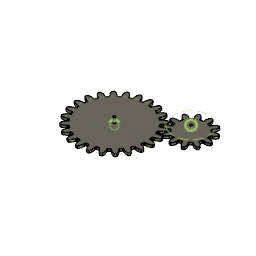
day5 joint and motion (Autodesk Fusion 360 design; units mm, degrees)
part number: 2026-04-16-20-59-54-327
description: Spur Gear; Module: 12.7; Num Teeth: 24; Pressure Angle: 20.0; Backlash: 0.00 mm
part number: 2026-04-16-21-00-13-750
description: Spur Gear; Module: 12.7; Num Teeth: 12; Pressure Angle: 20.0; Backlash: 0.00 mm
part number: 2026-04-16-21-00-25-707
part number: 2026-04-16-21-14-06-063
Autodesk Fusion 360 part; units mm, degrees
(part 1 of 2)
sketch "Base Circle" plane through (0, 0, 0) normal (0, 0, 1) x (1, 0, 0) in component "Spur Gear 24 teeth"
  circle A0 centre (0, 0) radius 137.7061
  circle A1 centre (0, 0) radius 5
extrude "Extrude1" add sketch "Base Circle" along normal blind 10 makes body 1 in component "Spur Gear 24 teeth"
sketch "Gear Tooth" plane through (0, 0, 0) normal (0, 0, 1) x (1, 0, 0) in component "Spur Gear 24 teeth"
  spline S0 degree 5 poles (142.7471, -11.4951) (142.8118, -11.5003) (142.9412, -11.5091) (143.1354, -11.5173) (143.3946, -11.5189) (143.7188, -11.5082) (144.0432, -11.4883) (144.3678, -11.4628) (144.6924, -11.4343) (145.0169, -11.4038) (145.3415, -11.3711) (145.666, -11.3355) (145.9905, -11.2961) (146.3148, -11.2522) (146.6391, -11.2039) (146.9633, -11.1516) (147.2873, -11.0957) (147.6112, -11.037) (147.935, -10.9757) (148.2586, -10.9121) (148.5821, -10.846) (148.9053, -10.7774) (149.2285, -10.7062) (149.5514, -10.6322) (149.8741, -10.5555) (150.1966, -10.4762) (150.5189, -10.3945) (150.8411, -10.3105) (151.1629, -10.2242) (151.4846, -10.1358) (151.806, -10.0451) (152.1272, -9.9523) (152.4482, -9.8574) (152.7689, -9.7602) (153.0893, -9.661) (153.4095, -9.5596) (153.7295, -9.4562) (154.0491, -9.3508) (154.3685, -9.2434) (154.6877, -9.1341) (155.0065, -9.0228) (155.325, -8.9096) (155.6433, -8.7946) (155.9613, -8.6776) (156.279, -8.5588) (156.5963, -8.4382) (156.9134, -8.3157) (157.2301, -8.1914) (157.5466, -8.0654) (157.8627, -7.9376) (158.1785, -7.808) (158.494, -7.6767) (158.8091, -7.5437) (159.1239, -7.409) (159.4384, -7.2727) (159.7525, -7.1346) (160.0663, -6.9949) (160.3798, -6.8535) (160.6929, -6.7105) (161.0056, -6.5659) (161.318, -6.4196) (161.63, -6.2718) (161.9417, -6.1224) (162.253, -5.9714) (162.5639, -5.8189) (162.8745, -5.6648) (163.1846, -5.5091) (163.4944, -5.352) (163.8038, -5.1933) (164.1128, -5.0331) (164.4215, -4.8714) (164.6681, -4.7409) (164.8528, -4.6423) (164.9759, -4.5763) (165.0375, -4.5432) knots 0 0 0 0 0 0 0.01428571 0.02857143 0.04285714 0.05714286 0.07142857 0.08571429 0.1 0.11428571 0.12857143 0.14285714 0.15714286 0.17142857 0.18571429 0.2 0.21428571 0.22857143 0.24285714 0.25714286 0.27142857 0.28571429 0.3 0.31428571 0.32857143 0.34285714 0.35714286 0.37142857 0.38571429 0.4 0.41428571 0.42857143 0.44285714 0.45714286 0.47142857 0.48571429 0.5 0.51428571 0.52857143 0.54285714 0.55714286 0.57142857 0.58571429 0.6 0.61428571 0.62857143 0.64285714 0.65714286 0.67142857 0.68571429 0.7 0.71428571 0.72857143 0.74285714 0.75714286 0.77142857 0.78571429 0.8 0.81428571 0.82857143 0.84285714 0.85714286 0.87142857 0.88571429 0.9 0.91428571 0.92857143 0.94285714 0.95714286 0.97142857 0.98571429 1 1 1 1 1 1
  spline S1 degree 5 poles (142.7471, 11.4951) (142.8118, 11.5003) (142.9412, 11.5091) (143.1354, 11.5173) (143.3946, 11.5189) (143.7188, 11.5082) (144.0432, 11.4883) (144.3678, 11.4628) (144.6924, 11.4343) (145.0169, 11.4038) (145.3415, 11.3711) (145.666, 11.3355) (145.9905, 11.2961) (146.3148, 11.2522) (146.6391, 11.2039) (146.9633, 11.1516) (147.2873, 11.0957) (147.6112, 11.037) (147.935, 10.9757) (148.2586, 10.9121) (148.5821, 10.846) (148.9053, 10.7774) (149.2285, 10.7062) (149.5514, 10.6322) (149.8741, 10.5555) (150.1966, 10.4762) (150.5189, 10.3945) (150.8411, 10.3105) (151.1629, 10.2242) (151.4846, 10.1358) (151.806, 10.0451) (152.1272, 9.9523) (152.4482, 9.8574) (152.7689, 9.7602) (153.0893, 9.661) (153.4095, 9.5596) (153.7295, 9.4562) (154.0491, 9.3508) (154.3685, 9.2434) (154.6877, 9.1341) (155.0065, 9.0228) (155.325, 8.9096) (155.6433, 8.7946) (155.9613, 8.6776) (156.279, 8.5588) (156.5963, 8.4382) (156.9134, 8.3157) (157.2301, 8.1914) (157.5466, 8.0654) (157.8627, 7.9376) (158.1785, 7.808) (158.494, 7.6767) (158.8091, 7.5437) (159.1239, 7.409) (159.4384, 7.2727) (159.7525, 7.1346) (160.0663, 6.9949) (160.3798, 6.8535) (160.6929, 6.7105) (161.0056, 6.5659) (161.318, 6.4196) (161.63, 6.2718) (161.9417, 6.1224) (162.253, 5.9714) (162.5639, 5.8189) (162.8745, 5.6648) (163.1846, 5.5091) (163.4944, 5.352) (163.8038, 5.1933) (164.1128, 5.0331) (164.4215, 4.8714) (164.6681, 4.7409) (164.8528, 4.6423) (164.9759, 4.5763) (165.0375, 4.5432) knots 0 0 0 0 0 0 0.01428571 0.02857143 0.04285714 0.05714286 0.07142857 0.08571429 0.1 0.11428571 0.12857143 0.14285714 0.15714286 0.17142857 0.18571429 0.2 0.21428571 0.22857143 0.24285714 0.25714286 0.27142857 0.28571429 0.3 0.31428571 0.32857143 0.34285714 0.35714286 0.37142857 0.38571429 0.4 0.41428571 0.42857143 0.44285714 0.45714286 0.47142857 0.48571429 0.5 0.51428571 0.52857143 0.54285714 0.55714286 0.57142857 0.58571429 0.6 0.61428571 0.62857143 0.64285714 0.65714286 0.67142857 0.68571429 0.7 0.71428571 0.72857143 0.74285714 0.75714286 0.77142857 0.78571429 0.8 0.81428571 0.82857143 0.84285714 0.85714286 0.87142857 0.88571429 0.9 0.91428571 0.92857143 0.94285714 0.95714286 0.97142857 0.98571429 1 1 1 1 1 1
  arc A0 (165.0375, -4.5432) -> (165.0375, 4.5432) centre (0, 0) ccw
  line L0 (137.2518, -11.0526) -> (142.7471, -11.4951)
  line L1 (137.2518, 11.0526) -> (142.7471, 11.4951)
  line L2 (137.2518, -11.0526) -> (137.2518, 11.0526)
  point P0 (144.318, -11.4661)
  point P1 (145.899, -11.3066)
  point P2 (147.486, -11.0593)
  point P3 (149.0774, -10.7392)
  point P4 (150.672, -10.3543)
  point P5 (152.2688, -9.9102)
  point P6 (153.8671, -9.4106)
  point P7 (155.466, -8.8584)
  point P8 (157.065, -8.256)
  point P9 (158.6633, -7.605)
  point P10 (160.2603, -6.9071)
  point P11 (161.8554, -6.1635)
  point P12 (163.448, -5.3752)
  point P13 (144.318, 11.4661)
  point P14 (145.899, 11.3066)
  point P15 (147.486, 11.0593)
  point P16 (149.0774, 10.7392)
  point P17 (150.672, 10.3543)
  point P18 (152.2688, 9.9102)
  point P19 (153.8671, 9.4106)
  point P20 (155.466, 8.8584)
  point P21 (157.065, 8.256)
  point P22 (158.6633, 7.605)
  point P23 (160.2603, 6.9071)
  point P24 (161.8554, 6.1635)
  point P25 (163.448, 5.3752)
extrude "Extrude2" add sketch "Gear Tooth" along normal blind 10 bodies 1 in component "Spur Gear 24 teeth"
fillet "Fillet1" radius 2 2 edges at (137.2618, -11.0534, 5) (137.2618, 11.0534, 5) on bodies 1 in component "Spur Gear 24 teeth"
pattern_circular "C-Pattern1" count 24 over 360 about axis through (0, 0, 0) along (0, 0, 1) of "Extrude2", "Fillet1" in component "Spur Gear 24 teeth"
sketch "Diametrial Pitch Circle" plane through (0, 0, 0) normal (0, 0, 1) x (1, 0, 0) in component "Spur Gear 24 teeth"
  circle A0 centre (0, 0) radius 152.4 construction
sketch "Base Circle (2)" plane through (0, 0, 0) normal (0, 0, 1) x (1, 0, 0) in component "Spur Gear 12 teeth"
  circle A0 centre (0, 0) radius 61.5061
  circle A1 centre (0, 0) radius 5
extrude "Extrude1'" add sketch "Base Circle (2)" along normal blind 10 separate body makes body 2 in component "Spur Gear 12 teeth"
sketch "Gear Tooth (2)" plane through (0, 0, 0) normal (0, 0, 1) x (1, 0, 0) in component "Spur Gear 12 teeth"
  spline S0 degree 5 poles (70.8448, -10.4033) (70.8965, -10.4109) (71.0001, -10.4244) (71.1558, -10.4396) (71.3641, -10.4502) (71.6254, -10.4506) (71.8873, -10.4416) (72.1496, -10.4272) (72.4121, -10.4097) (72.6748, -10.3901) (72.9374, -10.3683) (73.2002, -10.3433) (73.463, -10.3142) (73.726, -10.2804) (73.989, -10.2421) (74.2521, -10.1996) (74.5151, -10.1535) (74.7781, -10.1045) (75.041, -10.0529) (75.3037, -9.9989) (75.5664, -9.9422) (75.8289, -9.8828) (76.0913, -9.8206) (76.3536, -9.7555) (76.6157, -9.6876) (76.8776, -9.6169) (77.1394, -9.5437) (77.4009, -9.4681) (77.6622, -9.3901) (77.9233, -9.3098) (78.1842, -9.2272) (78.4448, -9.1423) (78.7051, -9.055) (78.9652, -8.9654) (79.225, -8.8736) (79.4846, -8.7796) (79.7438, -8.6834) (80.0027, -8.585) (80.2613, -8.4845) (80.5196, -8.382) (80.7775, -8.2774) (81.0352, -8.1707) (81.2924, -8.062) (81.5493, -7.9513) (81.8059, -7.8386) (82.0621, -7.7239) (82.3179, -7.6073) (82.5733, -7.4887) (82.8283, -7.3682) (83.0829, -7.2459) (83.3371, -7.1216) (83.5909, -6.9955) (83.8443, -6.8676) (84.0972, -6.7378) (84.3497, -6.6062) (84.6018, -6.4728) (84.8534, -6.3376) (85.1045, -6.2006) (85.3552, -6.0619) (85.6054, -5.9214) (85.8552, -5.7792) (86.1044, -5.6353) (86.3532, -5.4897) (86.6015, -5.3423) (86.8493, -5.1933) (87.0965, -5.0426) (87.3433, -4.8902) (87.5895, -4.7362) (87.8352, -4.5806) (88.0804, -4.4233) (88.325, -4.2644) (88.5203, -4.136) (88.6665, -4.039) (88.7639, -3.974) (88.8126, -3.9414) knots 0 0 0 0 0 0 0.01428571 0.02857143 0.04285714 0.05714286 0.07142857 0.08571429 0.1 0.11428571 0.12857143 0.14285714 0.15714286 0.17142857 0.18571429 0.2 0.21428571 0.22857143 0.24285714 0.25714286 0.27142857 0.28571429 0.3 0.31428571 0.32857143 0.34285714 0.35714286 0.37142857 0.38571429 0.4 0.41428571 0.42857143 0.44285714 0.45714286 0.47142857 0.48571429 0.5 0.51428571 0.52857143 0.54285714 0.55714286 0.57142857 0.58571429 0.6 0.61428571 0.62857143 0.64285714 0.65714286 0.67142857 0.68571429 0.7 0.71428571 0.72857143 0.74285714 0.75714286 0.77142857 0.78571429 0.8 0.81428571 0.82857143 0.84285714 0.85714286 0.87142857 0.88571429 0.9 0.91428571 0.92857143 0.94285714 0.95714286 0.97142857 0.98571429 1 1 1 1 1 1
  spline S1 degree 5 poles (70.8448, 10.4033) (70.8965, 10.4109) (71.0001, 10.4244) (71.1558, 10.4396) (71.3641, 10.4502) (71.6254, 10.4506) (71.8873, 10.4416) (72.1496, 10.4272) (72.4121, 10.4097) (72.6748, 10.3901) (72.9374, 10.3683) (73.2002, 10.3433) (73.463, 10.3142) (73.726, 10.2804) (73.989, 10.2421) (74.2521, 10.1996) (74.5151, 10.1535) (74.7781, 10.1045) (75.041, 10.0529) (75.3037, 9.9989) (75.5664, 9.9422) (75.8289, 9.8828) (76.0913, 9.8206) (76.3536, 9.7555) (76.6157, 9.6876) (76.8776, 9.6169) (77.1394, 9.5437) (77.4009, 9.4681) (77.6622, 9.3901) (77.9233, 9.3098) (78.1842, 9.2272) (78.4448, 9.1423) (78.7051, 9.055) (78.9652, 8.9654) (79.225, 8.8736) (79.4846, 8.7796) (79.7438, 8.6834) (80.0027, 8.585) (80.2613, 8.4845) (80.5196, 8.382) (80.7775, 8.2774) (81.0352, 8.1707) (81.2924, 8.062) (81.5493, 7.9513) (81.8059, 7.8386) (82.0621, 7.7239) (82.3179, 7.6073) (82.5733, 7.4887) (82.8283, 7.3682) (83.0829, 7.2459) (83.3371, 7.1216) (83.5909, 6.9955) (83.8443, 6.8676) (84.0972, 6.7378) (84.3497, 6.6062) (84.6018, 6.4728) (84.8534, 6.3376) (85.1045, 6.2006) (85.3552, 6.0619) (85.6054, 5.9214) (85.8552, 5.7792) (86.1044, 5.6353) (86.3532, 5.4897) (86.6015, 5.3423) (86.8493, 5.1933) (87.0965, 5.0426) (87.3433, 4.8902) (87.5895, 4.7362) (87.8352, 4.5806) (88.0804, 4.4233) (88.325, 4.2644) (88.5203, 4.136) (88.6665, 4.039) (88.7639, 3.974) (88.8126, 3.9414) knots 0 0 0 0 0 0 0.01428571 0.02857143 0.04285714 0.05714286 0.07142857 0.08571429 0.1 0.11428571 0.12857143 0.14285714 0.15714286 0.17142857 0.18571429 0.2 0.21428571 0.22857143 0.24285714 0.25714286 0.27142857 0.28571429 0.3 0.31428571 0.32857143 0.34285714 0.35714286 0.37142857 0.38571429 0.4 0.41428571 0.42857143 0.44285714 0.45714286 0.47142857 0.48571429 0.5 0.51428571 0.52857143 0.54285714 0.55714286 0.57142857 0.58571429 0.6 0.61428571 0.62857143 0.64285714 0.65714286 0.67142857 0.68571429 0.7 0.71428571 0.72857143 0.74285714 0.75714286 0.77142857 0.78571429 0.8 0.81428571 0.82857143 0.84285714 0.85714286 0.87142857 0.88571429 0.9 0.91428571 0.92857143 0.94285714 0.95714286 0.97142857 0.98571429 1 1 1 1 1 1
  arc A0 (88.8126, -3.9414) -> (88.8126, 3.9414) centre (0, 0) ccw
  line L0 (60.8436, -8.9346) -> (70.8448, -10.4033)
  line L1 (60.8436, 8.9346) -> (70.8448, 10.4033)
  line L2 (60.8436, -8.9346) -> (60.8436, 8.9346)
  point P0 (72.0894, -10.43)
  point P1 (73.3521, -10.3259)
  point P2 (74.626, -10.1325)
  point P3 (75.908, -9.8637)
  point P4 (77.1959, -9.527)
  point P5 (78.488, -9.1273)
  point P6 (79.7828, -8.6681)
  point P7 (81.0789, -8.1518)
  point P8 (82.375, -7.5804)
  point P9 (83.6699, -6.9554)
  point P10 (84.9622, -6.278)
  point P11 (86.2509, -5.5493)
  point P12 (87.5347, -4.7702)
  point P13 (72.0894, 10.43)
  point P14 (73.3521, 10.3259)
  point P15 (74.626, 10.1325)
  point P16 (75.908, 9.8637)
  point P17 (77.1959, 9.527)
  point P18 (78.488, 9.1273)
  point P19 (79.7828, 8.6681)
  point P20 (81.0789, 8.1518)
  point P21 (82.375, 7.5804)
  point P22 (83.6699, 6.9554)
  point P23 (84.9622, 6.278)
  point P24 (86.2509, 5.5493)
  point P25 (87.5347, 4.7702)
extrude "Extrude2'" add sketch "Gear Tooth (2)" along normal blind 10 bodies 2 in component "Spur Gear 12 teeth"
fillet "Fillet1'" radius 2 2 edges at (60.8535, -8.9361, 5) (60.8535, 8.9361, 5) on bodies 2 in component "Spur Gear 12 teeth"
pattern_circular "C-Pattern1'" count 12 over 360 about axis through (0, 0, 0) along (0, 0, 1) of "Extrude2'", "Fillet1'" in component "Spur Gear 12 teeth"
sketch "Diametrial Pitch Circle (2)" plane through (0, 0, 0) normal (0, 0, 1) x (1, 0, 0) in component "Spur Gear 12 teeth"
  circle A0 centre (0, 0) radius 76.2 construction
sketch "Sketch1" plane through (0, 0, 0) normal (0, 0, 1) x (-0.5, -0.866025, 0)
  circle A0 centre (0, 0) radius 5
  dimension "d17" = 10
  constraint coincident A0.centre origin
  measures "d17" diameter of A0
extrude "Extrude3" add sketch "Sketch1" along normal blind 31.7 and the other way blind 20 sketch seen with x (-0.5, 0.866025, 0) y (-0.866025, -0.5, 0) z (0, 0, 1) at (0, 0, 0) bodies 1 in component "Spur Gear 24 teeth"
sketch "Sketch2" plane through (0, 0, 7.8995) normal (0, 0, 1) x (-1, 0, 0)
  arc A0 (-143.633, -92.0504) -> (-150.974, -84.7093) centre (-190.6397, -131.7161) ccw
  arc A1 (-151.2526, -81.9398) -> (-150.974, -84.7093) centre (-149.6842, -83.1808) ccw
  line L0 (-151.2526, -81.9398) -> (-146.2078, -75.5643)
  spline S0 degree 5 poles (-146.2078, -75.5643) (-146.1754, -75.5233) (-146.1119, -75.4404) (-146.0209, -75.3131) (-145.9075, -75.1381) (-145.7766, -74.912) (-145.6533, -74.6807) (-145.5347, -74.4462) (-145.4186, -74.2102) (-145.3042, -73.9729) (-145.1918, -73.7345) (-145.0821, -73.4945) (-144.9759, -73.2523) (-144.8736, -73.0077) (-144.7753, -72.7608) (-144.6806, -72.5117) (-144.589, -72.2609) (-144.4999, -72.0086) (-144.4131, -71.7552) (-144.3286, -71.5006) (-144.2463, -71.2448) (-144.1665, -70.9877) (-144.0892, -70.7294) (-144.0144, -70.4697) (-143.9422, -70.2087) (-143.8724, -69.9466) (-143.8049, -69.6833) (-143.7396, -69.419) (-143.6765, -69.1537) (-143.6155, -68.8874) (-143.5566, -68.6202) (-143.4999, -68.352) (-143.4453, -68.0829) (-143.3928, -67.8129) (-143.3424, -67.542) (-143.2941, -67.2702) (-143.2478, -66.9976) (-143.2035, -66.7242) (-143.1612, -66.45) (-143.1209, -66.175) (-143.0825, -65.8993) (-143.0461, -65.6229) (-143.0116, -65.3458) (-142.979, -65.0679) (-142.9484, -64.7894) (-142.9196, -64.5102) (-142.8927, -64.2303) (-142.8677, -63.9499) (-142.8445, -63.6688) (-142.8232, -63.3871) (-142.8036, -63.1048) (-142.786, -62.822) (-142.7701, -62.5386) (-142.756, -62.2547) (-142.7437, -61.9702) (-142.7332, -61.6852) (-142.7245, -61.3997) (-142.7176, -61.1137) (-142.7124, -60.8273) (-142.7089, -60.5403) (-142.7072, -60.2529) (-142.7072, -59.9651) (-142.7089, -59.6768) (-142.7124, -59.3882) (-142.7176, -59.0991) (-142.7244, -58.8096) (-142.733, -58.5197) (-142.7433, -58.2295) (-142.7552, -57.9388) (-142.7688, -57.6479) (-142.7841, -57.3566) (-142.7976, -57.1232) (-142.8086, -56.9481) (-142.8162, -56.8313) (-142.8201, -56.7728) knots 0 0 0 0 0 0 0.01428571 0.02857143 0.04285714 0.05714286 0.07142857 0.08571429 0.1 0.11428571 0.12857143 0.14285714 0.15714286 0.17142857 0.18571429 0.2 0.21428571 0.22857143 0.24285714 0.25714286 0.27142857 0.28571429 0.3 0.31428571 0.32857143 0.34285714 0.35714286 0.37142857 0.38571429 0.4 0.41428571 0.42857143 0.44285714 0.45714286 0.47142857 0.48571429 0.5 0.51428571 0.52857143 0.54285714 0.55714286 0.57142857 0.58571429 0.6 0.61428571 0.62857143 0.64285714 0.65714286 0.67142857 0.68571429 0.7 0.71428571 0.72857143 0.74285714 0.75714286 0.77142857 0.78571429 0.8 0.81428571 0.82857143 0.84285714 0.85714286 0.87142857 0.88571429 0.9 0.91428571 0.92857143 0.94285714 0.95714286 0.97142857 0.98571429 1 1 1 1 1 1
  arc A2 (-142.8201, -56.7728) -> (-149.6468, -52.8314) centre (-190.6397, -131.7161) ccw
  spline S1 degree 5 poles (-149.6468, -52.8314) (-149.6993, -52.8573) (-149.8043, -52.9091) (-149.9615, -52.9872) (-150.1703, -53.0921) (-150.4302, -53.2246) (-150.689, -53.3582) (-150.9467, -53.4932) (-151.2031, -53.6295) (-151.4585, -53.767) (-151.7126, -53.9058) (-151.9656, -54.0458) (-152.2173, -54.1872) (-152.4678, -54.3298) (-152.7171, -54.4737) (-152.9651, -54.6189) (-153.2119, -54.7653) (-153.4574, -54.9131) (-153.7016, -55.0621) (-153.9444, -55.2124) (-154.186, -55.364) (-154.4262, -55.5169) (-154.6651, -55.671) (-154.9026, -55.8265) (-155.1387, -55.9832) (-155.3734, -56.1412) (-155.6067, -56.3006) (-155.8385, -56.4612) (-156.0689, -56.6231) (-156.2978, -56.7863) (-156.5252, -56.9508) (-156.7511, -57.1166) (-156.9754, -57.2838) (-157.1982, -57.4522) (-157.4193, -57.622) (-157.6389, -57.7931) (-157.8569, -57.9655) (-158.0732, -58.1392) (-158.2878, -58.3143) (-158.5008, -58.4906) (-158.712, -58.6684) (-158.9214, -58.8475) (-159.129, -59.0279) (-159.3348, -59.2098) (-159.5386, -59.393) (-159.7406, -59.5776) (-159.9407, -59.7635) (-160.1389, -59.9509) (-160.3352, -60.1395) (-160.5294, -60.3296) (-160.7216, -60.5212) (-160.9114, -60.7142) (-161.099, -60.9087) (-161.284, -61.1049) (-161.4667, -61.3026) (-161.6471, -61.5017) (-161.8253, -61.7022) (-162.0015, -61.9041) (-162.1754, -62.1073) (-162.3468, -62.3121) (-162.5151, -62.5187) (-162.6798, -62.7273) (-162.8405, -62.9381) (-162.9972, -63.1512) (-163.1502, -63.3662) (-163.3005, -63.5828) (-163.4487, -63.8005) (-163.5951, -64.0191) (-163.7388, -64.239) (-163.8775, -64.4614) (-164.0079, -64.6878) (-164.1028, -64.8735) (-164.1675, -65.016) (-164.2075, -65.1124) (-164.2268, -65.161) knots -1 -1 -1 -1 -1 -1 -0.98571429 -0.97142857 -0.95714286 -0.94285714 -0.92857143 -0.91428571 -0.9 -0.88571429 -0.87142857 -0.85714286 -0.84285714 -0.82857143 -0.81428571 -0.8 -0.78571429 -0.77142857 -0.75714286 -0.74285714 -0.72857143 -0.71428571 -0.7 -0.68571429 -0.67142857 -0.65714286 -0.64285714 -0.62857143 -0.61428571 -0.6 -0.58571429 -0.57142857 -0.55714286 -0.54285714 -0.52857143 -0.51428571 -0.5 -0.48571429 -0.47142857 -0.45714286 -0.44285714 -0.42857143 -0.41428571 -0.4 -0.38571429 -0.37142857 -0.35714286 -0.34285714 -0.32857143 -0.31428571 -0.3 -0.28571429 -0.27142857 -0.25714286 -0.24285714 -0.22857143 -0.21428571 -0.2 -0.18571429 -0.17142857 -0.15714286 -0.14285714 -0.12857143 -0.11428571 -0.1 -0.08571429 -0.07142857 -0.05714286 -0.04285714 -0.02857143 -0.01428571 0 0 0 0 0 0
  line L1 (-164.2268, -65.161) -> (-167.2257, -72.7177)
  arc A3 (-169.7635, -73.8612) -> (-167.2257, -72.7177) centre (-169.0847, -71.9799) ccw
  arc A4 (-169.7635, -73.8612) -> (-179.7916, -71.1742) centre (-190.6397, -131.7161) ccw
  arc A5 (-181.4176, -68.915) -> (-179.7916, -71.1742) centre (-179.4388, -69.2055) ccw
  line L2 (-181.4176, -68.915) -> (-180.2364, -60.8713)
  spline S2 degree 5 poles (-180.2364, -60.8713) (-180.2288, -60.8195) (-180.2153, -60.716) (-180.2001, -60.5603) (-180.1895, -60.352) (-180.1891, -60.0907) (-180.1981, -59.8288) (-180.2125, -59.5664) (-180.23, -59.3039) (-180.2496, -59.0413) (-180.2714, -58.7786) (-180.2964, -58.5159) (-180.3255, -58.253) (-180.3593, -57.9901) (-180.3976, -57.7271) (-180.4401, -57.464) (-180.4862, -57.201) (-180.5352, -56.938) (-180.5868, -56.6751) (-180.6409, -56.4123) (-180.6975, -56.1497) (-180.7569, -55.8872) (-180.8191, -55.6248) (-180.8842, -55.3625) (-180.9521, -55.1004) (-181.0228, -54.8385) (-181.096, -54.5767) (-181.1716, -54.3152) (-181.2496, -54.0538) (-181.3299, -53.7927) (-181.4125, -53.5319) (-181.4975, -53.2713) (-181.5847, -53.0109) (-181.6743, -52.7509) (-181.7661, -52.491) (-181.8601, -52.2315) (-181.9564, -51.9723) (-182.0547, -51.7134) (-182.1552, -51.4548) (-182.2577, -51.1965) (-182.3624, -50.9385) (-182.469, -50.6809) (-182.5777, -50.4236) (-182.6884, -50.1667) (-182.8011, -49.9102) (-182.9158, -49.654) (-183.0324, -49.3982) (-183.151, -49.1428) (-183.2715, -48.8878) (-183.3938, -48.6332) (-183.5181, -48.379) (-183.6442, -48.1252) (-183.7721, -47.8718) (-183.9019, -47.6189) (-184.0335, -47.3664) (-184.1669, -47.1143) (-184.3021, -46.8627) (-184.4391, -46.6116) (-184.5778, -46.3609) (-184.7183, -46.1107) (-184.8605, -45.8609) (-185.0044, -45.6117) (-185.1501, -45.3629) (-185.2974, -45.1146) (-185.4464, -44.8668) (-185.5971, -44.6195) (-185.7495, -44.3728) (-185.9035, -44.1266) (-186.0591, -43.8809) (-186.2164, -43.6357) (-186.3753, -43.391) (-186.5037, -43.1958) (-186.6007, -43.0495) (-186.6657, -42.9521) (-186.6983, -42.9035) knots 0 0 0 0 0 0 0.01428571 0.02857143 0.04285714 0.05714286 0.07142857 0.08571429 0.1 0.11428571 0.12857143 0.14285714 0.15714286 0.17142857 0.18571429 0.2 0.21428571 0.22857143 0.24285714 0.25714286 0.27142857 0.28571429 0.3 0.31428571 0.32857143 0.34285714 0.35714286 0.37142857 0.38571429 0.4 0.41428571 0.42857143 0.44285714 0.45714286 0.47142857 0.48571429 0.5 0.51428571 0.52857143 0.54285714 0.55714286 0.57142857 0.58571429 0.6 0.61428571 0.62857143 0.64285714 0.65714286 0.67142857 0.68571429 0.7 0.71428571 0.72857143 0.74285714 0.75714286 0.77142857 0.78571429 0.8 0.81428571 0.82857143 0.84285714 0.85714286 0.87142857 0.88571429 0.9 0.91428571 0.92857143 0.94285714 0.95714286 0.97142857 0.98571429 1 1 1 1 1 1
  arc A6 (-186.6983, -42.9035) -> (-194.5811, -42.9035) centre (-190.6397, -131.7161) ccw
  spline S3 degree 5 poles (-194.5811, -42.9035) (-194.6137, -42.9521) (-194.6787, -43.0495) (-194.7758, -43.1958) (-194.9042, -43.391) (-195.063, -43.6357) (-195.2203, -43.8809) (-195.376, -44.1266) (-195.53, -44.3728) (-195.6823, -44.6195) (-195.833, -44.8668) (-195.982, -45.1146) (-196.1294, -45.3629) (-196.275, -45.6117) (-196.4189, -45.8609) (-196.5611, -46.1107) (-196.7016, -46.3609) (-196.8403, -46.6116) (-196.9773, -46.8627) (-197.1125, -47.1143) (-197.2459, -47.3664) (-197.3775, -47.6189) (-197.5073, -47.8718) (-197.6352, -48.1252) (-197.7613, -48.379) (-197.8856, -48.6332) (-198.008, -48.8878) (-198.1284, -49.1428) (-198.247, -49.3982) (-198.3636, -49.654) (-198.4783, -49.9102) (-198.591, -50.1667) (-198.7017, -50.4236) (-198.8104, -50.6809) (-198.9171, -50.9385) (-199.0217, -51.1965) (-199.1242, -51.4548) (-199.2247, -51.7134) (-199.3231, -51.9723) (-199.4193, -52.2315) (-199.5133, -52.491) (-199.6052, -52.7509) (-199.6947, -53.0109) (-199.782, -53.2713) (-199.8669, -53.5319) (-199.9495, -53.7927) (-200.0298, -54.0538) (-200.1078, -54.3152) (-200.1835, -54.5767) (-200.2567, -54.8385) (-200.3273, -55.1004) (-200.3952, -55.3625) (-200.4603, -55.6248) (-200.5225, -55.8872) (-200.5819, -56.1497) (-200.6386, -56.4123) (-200.6927, -56.6751) (-200.7443, -56.938) (-200.7932, -57.201) (-200.8393, -57.464) (-200.8818, -57.7271) (-200.9201, -57.9901) (-200.9539, -58.253) (-200.983, -58.5159) (-201.008, -58.7786) (-201.0299, -59.0413) (-201.0494, -59.3039) (-201.0669, -59.5664) (-201.0814, -59.8288) (-201.0903, -60.0907) (-201.09, -60.352) (-201.0793, -60.5603) (-201.0641, -60.716) (-201.0506, -60.8195) (-201.043, -60.8713) knots -1 -1 -1 -1 -1 -1 -0.98571429 -0.97142857 -0.95714286 -0.94285714 -0.92857143 -0.91428571 -0.9 -0.88571429 -0.87142857 -0.85714286 -0.84285714 -0.82857143 -0.81428571 -0.8 -0.78571429 -0.77142857 -0.75714286 -0.74285714 -0.72857143 -0.71428571 -0.7 -0.68571429 -0.67142857 -0.65714286 -0.64285714 -0.62857143 -0.61428571 -0.6 -0.58571429 -0.57142857 -0.55714286 -0.54285714 -0.52857143 -0.51428571 -0.5 -0.48571429 -0.47142857 -0.45714286 -0.44285714 -0.42857143 -0.41428571 -0.4 -0.38571429 -0.37142857 -0.35714286 -0.34285714 -0.32857143 -0.31428571 -0.3 -0.28571429 -0.27142857 -0.25714286 -0.24285714 -0.22857143 -0.21428571 -0.2 -0.18571429 -0.17142857 -0.15714286 -0.14285714 -0.12857143 -0.11428571 -0.1 -0.08571429 -0.07142857 -0.05714286 -0.04285714 -0.02857143 -0.01428571 0 0 0 0 0 0
  line L3 (-201.043, -60.8713) -> (-199.8618, -68.915)
  arc A7 (-201.4878, -71.1742) -> (-199.8618, -68.915) centre (-201.8406, -69.2055) ccw
  arc A8 (-201.4878, -71.1742) -> (-211.5159, -73.8612) centre (-190.6397, -131.7161) ccw
  arc A9 (-214.0537, -72.7177) -> (-211.5159, -73.8612) centre (-212.1947, -71.9799) ccw
  line L4 (-214.0537, -72.7177) -> (-217.0526, -65.161)
  spline S4 degree 5 poles (-217.0526, -65.161) (-217.0719, -65.1124) (-217.112, -65.016) (-217.1767, -64.8735) (-217.2716, -64.6878) (-217.4019, -64.4614) (-217.5406, -64.239) (-217.6843, -64.0191) (-217.8307, -63.8005) (-217.979, -63.5828) (-218.1292, -63.3662) (-218.2823, -63.1512) (-218.4389, -62.9381) (-218.5996, -62.7273) (-218.7643, -62.5187) (-218.9326, -62.3121) (-219.104, -62.1073) (-219.278, -61.9041) (-219.4541, -61.7022) (-219.6323, -61.5017) (-219.8127, -61.3026) (-219.9954, -61.1049) (-220.1805, -60.9087) (-220.368, -60.7142) (-220.5579, -60.5212) (-220.75, -60.3296) (-220.9443, -60.1395) (-221.1405, -59.9509) (-221.3387, -59.7635) (-221.5388, -59.5776) (-221.7408, -59.393) (-221.9447, -59.2098) (-222.1504, -59.0279) (-222.358, -58.8475) (-222.5674, -58.6684) (-222.7786, -58.4906) (-222.9916, -58.3143) (-223.2062, -58.1392) (-223.4226, -57.9655) (-223.6405, -57.7931) (-223.8601, -57.622) (-224.0813, -57.4522) (-224.304, -57.2838) (-224.5284, -57.1166) (-224.7543, -56.9508) (-224.9817, -56.7863) (-225.2106, -56.6231) (-225.4409, -56.4612) (-225.6728, -56.3006) (-225.9061, -56.1412) (-226.1408, -55.9832) (-226.3769, -55.8265) (-226.6143, -55.671) (-226.8532, -55.5169) (-227.0934, -55.364) (-227.335, -55.2124) (-227.5779, -55.0621) (-227.8221, -54.9131) (-228.0675, -54.7653) (-228.3143, -54.6189) (-228.5623, -54.4737) (-228.8116, -54.3298) (-229.0621, -54.1872) (-229.3139, -54.0458) (-229.5668, -53.9058) (-229.821, -53.767) (-230.0763, -53.6295) (-230.3328, -53.4932) (-230.5904, -53.3582) (-230.8492, -53.2246) (-231.1091, -53.0921) (-231.318, -52.9872) (-231.4751, -52.9091) (-231.5801, -52.8573) (-231.6326, -52.8314) knots 0 0 0 0 0 0 0.01428571 0.02857143 0.04285714 0.05714286 0.07142857 0.08571429 0.1 0.11428571 0.12857143 0.14285714 0.15714286 0.17142857 0.18571429 0.2 0.21428571 0.22857143 0.24285714 0.25714286 0.27142857 0.28571429 0.3 0.31428571 0.32857143 0.34285714 0.35714286 0.37142857 0.38571429 0.4 0.41428571 0.42857143 0.44285714 0.45714286 0.47142857 0.48571429 0.5 0.51428571 0.52857143 0.54285714 0.55714286 0.57142857 0.58571429 0.6 0.61428571 0.62857143 0.64285714 0.65714286 0.67142857 0.68571429 0.7 0.71428571 0.72857143 0.74285714 0.75714286 0.77142857 0.78571429 0.8 0.81428571 0.82857143 0.84285714 0.85714286 0.87142857 0.88571429 0.9 0.91428571 0.92857143 0.94285714 0.95714286 0.97142857 0.98571429 1 1 1 1 1 1
  arc A10 (-231.6326, -52.8314) -> (-238.4594, -56.7728) centre (-190.6397, -131.7161) ccw
  spline S5 degree 5 poles (-238.4594, -56.7728) (-238.4633, -56.8313) (-238.4709, -56.9481) (-238.4818, -57.1232) (-238.4953, -57.3566) (-238.5106, -57.6479) (-238.5242, -57.9388) (-238.5362, -58.2295) (-238.5464, -58.5197) (-238.555, -58.8096) (-238.5619, -59.0991) (-238.567, -59.3882) (-238.5705, -59.6768) (-238.5722, -59.9651) (-238.5722, -60.2529) (-238.5705, -60.5403) (-238.5671, -60.8273) (-238.5619, -61.1137) (-238.5549, -61.3997) (-238.5462, -61.6852) (-238.5357, -61.9702) (-238.5234, -62.2547) (-238.5093, -62.5386) (-238.4935, -62.822) (-238.4758, -63.1048) (-238.4563, -63.3871) (-238.4349, -63.6688) (-238.4118, -63.9499) (-238.3867, -64.2303) (-238.3598, -64.5102) (-238.3311, -64.7894) (-238.3004, -65.0679) (-238.2678, -65.3458) (-238.2333, -65.6229) (-238.1969, -65.8993) (-238.1585, -66.175) (-238.1182, -66.45) (-238.0759, -66.7242) (-238.0316, -66.9976) (-237.9853, -67.2702) (-237.937, -67.542) (-237.8866, -67.8129) (-237.8341, -68.0829) (-237.7795, -68.352) (-237.7228, -68.6202) (-237.6639, -68.8874) (-237.6029, -69.1537) (-237.5398, -69.419) (-237.4745, -69.6833) (-237.407, -69.9466) (-237.3372, -70.2087) (-237.265, -70.4697) (-237.1903, -70.7294) (-237.113, -70.9877) (-237.0331, -71.2448) (-236.9508, -71.5006) (-236.8663, -71.7552) (-236.7795, -72.0086) (-236.6905, -72.2609) (-236.5988, -72.5117) (-236.5041, -72.7608) (-236.4058, -73.0077) (-236.3036, -73.2523) (-236.1974, -73.4945) (-236.0876, -73.7345) (-235.9752, -73.9729) (-235.8609, -74.2102) (-235.7447, -74.4462) (-235.6261, -74.6807) (-235.5028, -74.912) (-235.3719, -75.1381) (-235.2586, -75.3131) (-235.1675, -75.4404) (-235.1041, -75.5233) (-235.0716, -75.5643) knots -1 -1 -1 -1 -1 -1 -0.98571429 -0.97142857 -0.95714286 -0.94285714 -0.92857143 -0.91428571 -0.9 -0.88571429 -0.87142857 -0.85714286 -0.84285714 -0.82857143 -0.81428571 -0.8 -0.78571429 -0.77142857 -0.75714286 -0.74285714 -0.72857143 -0.71428571 -0.7 -0.68571429 -0.67142857 -0.65714286 -0.64285714 -0.62857143 -0.61428571 -0.6 -0.58571429 -0.57142857 -0.55714286 -0.54285714 -0.52857143 -0.51428571 -0.5 -0.48571429 -0.47142857 -0.45714286 -0.44285714 -0.42857143 -0.41428571 -0.4 -0.38571429 -0.37142857 -0.35714286 -0.34285714 -0.32857143 -0.31428571 -0.3 -0.28571429 -0.27142857 -0.25714286 -0.24285714 -0.22857143 -0.21428571 -0.2 -0.18571429 -0.17142857 -0.15714286 -0.14285714 -0.12857143 -0.11428571 -0.1 -0.08571429 -0.07142857 -0.05714286 -0.04285714 -0.02857143 -0.01428571 0 0 0 0 0 0
  line L5 (-235.0716, -75.5643) -> (-230.0268, -81.9398)
  arc A11 (-230.3054, -84.7093) -> (-230.0268, -81.9398) centre (-231.5952, -83.1808) ccw
  arc A12 (-230.3054, -84.7093) -> (-237.6465, -92.0504) centre (-190.6397, -131.7161) ccw
  arc A13 (-240.416, -92.3289) -> (-237.6465, -92.0504) centre (-239.175, -90.7606) ccw
  line L6 (-240.416, -92.3289) -> (-246.7915, -87.2842)
  spline S6 degree 5 poles (-246.7915, -87.2842) (-246.8325, -87.2517) (-246.9154, -87.1882) (-247.0427, -87.0972) (-247.2177, -86.9839) (-247.4438, -86.8529) (-247.6751, -86.7297) (-247.9095, -86.6111) (-248.1456, -86.4949) (-248.3828, -86.3806) (-248.6213, -86.2681) (-248.8613, -86.1584) (-249.1035, -86.0522) (-249.3481, -85.95) (-249.595, -85.8517) (-249.8441, -85.7569) (-250.0949, -85.6653) (-250.3472, -85.5762) (-250.6006, -85.4895) (-250.8552, -85.4049) (-251.111, -85.3227) (-251.3681, -85.2428) (-251.6264, -85.1655) (-251.8861, -85.0908) (-252.1471, -85.0185) (-252.4092, -84.9487) (-252.6725, -84.8813) (-252.9368, -84.816) (-253.2021, -84.7529) (-253.4684, -84.6919) (-253.7356, -84.633) (-254.0038, -84.5763) (-254.2729, -84.5216) (-254.5429, -84.4692) (-254.8138, -84.4188) (-255.0856, -84.3705) (-255.3582, -84.3242) (-255.6316, -84.2799) (-255.9058, -84.2376) (-256.1807, -84.1973) (-256.4564, -84.1589) (-256.7329, -84.1225) (-257.01, -84.088) (-257.2879, -84.0554) (-257.5664, -84.0247) (-257.8456, -83.9959) (-258.1254, -83.9691) (-258.4059, -83.944) (-258.687, -83.9208) (-258.9687, -83.8995) (-259.2509, -83.88) (-259.5338, -83.8623) (-259.8172, -83.8464) (-260.1011, -83.8324) (-260.3856, -83.8201) (-260.6706, -83.8096) (-260.9561, -83.8009) (-261.2421, -83.7939) (-261.5285, -83.7887) (-261.8155, -83.7853) (-262.1028, -83.7835) (-262.3907, -83.7836) (-262.6789, -83.7853) (-262.9676, -83.7888) (-263.2567, -83.7939) (-263.5462, -83.8008) (-263.8361, -83.8094) (-264.1263, -83.8196) (-264.4169, -83.8315) (-264.7079, -83.8452) (-264.9992, -83.8604) (-265.2325, -83.874) (-265.4077, -83.8849) (-265.5245, -83.8925) (-265.583, -83.8964) knots 0 0 0 0 0 0 0.01428571 0.02857143 0.04285714 0.05714286 0.07142857 0.08571429 0.1 0.11428571 0.12857143 0.14285714 0.15714286 0.17142857 0.18571429 0.2 0.21428571 0.22857143 0.24285714 0.25714286 0.27142857 0.28571429 0.3 0.31428571 0.32857143 0.34285714 0.35714286 0.37142857 0.38571429 0.4 0.41428571 0.42857143 0.44285714 0.45714286 0.47142857 0.48571429 0.5 0.51428571 0.52857143 0.54285714 0.55714286 0.57142857 0.58571429 0.6 0.61428571 0.62857143 0.64285714 0.65714286 0.67142857 0.68571429 0.7 0.71428571 0.72857143 0.74285714 0.75714286 0.77142857 0.78571429 0.8 0.81428571 0.82857143 0.84285714 0.85714286 0.87142857 0.88571429 0.9 0.91428571 0.92857143 0.94285714 0.95714286 0.97142857 0.98571429 1 1 1 1 1 1
  arc A14 (-265.583, -83.8964) -> (-269.5244, -90.7231) centre (-190.6397, -131.7161) ccw
  spline S7 degree 5 poles (-269.5244, -90.7231) (-269.4985, -90.7757) (-269.4467, -90.8807) (-269.3686, -91.0378) (-269.2637, -91.2467) (-269.1312, -91.5066) (-268.9975, -91.7654) (-268.8626, -92.023) (-268.7263, -92.2795) (-268.5888, -92.5348) (-268.45, -92.789) (-268.3099, -93.0419) (-268.1686, -93.2937) (-268.026, -93.5442) (-267.8821, -93.7934) (-267.7369, -94.0415) (-267.5904, -94.2882) (-267.4427, -94.5337) (-267.2937, -94.7779) (-267.1434, -95.0208) (-266.9918, -95.2624) (-266.8389, -95.5026) (-266.6848, -95.7414) (-266.5293, -95.9789) (-266.3726, -96.215) (-266.2146, -96.4497) (-266.0552, -96.683) (-265.8946, -96.9148) (-265.7327, -97.1452) (-265.5695, -97.3741) (-265.405, -97.6015) (-265.2392, -97.8274) (-265.072, -98.0518) (-264.9036, -98.2745) (-264.7338, -98.4957) (-264.5627, -98.7153) (-264.3903, -98.9332) (-264.2166, -99.1495) (-264.0415, -99.3642) (-263.8651, -99.5771) (-263.6874, -99.7883) (-263.5083, -99.9978) (-263.3279, -100.2054) (-263.146, -100.4111) (-262.9628, -100.615) (-262.7782, -100.8169) (-262.5922, -101.017) (-262.4049, -101.2152) (-262.2162, -101.4115) (-262.0262, -101.6058) (-261.8346, -101.7979) (-261.6416, -101.9878) (-261.447, -102.1753) (-261.2509, -102.3604) (-261.0532, -102.5431) (-260.8541, -102.7235) (-260.6536, -102.9017) (-260.4517, -103.0778) (-260.2484, -103.2517) (-260.0437, -103.4231) (-259.8371, -103.5915) (-259.6285, -103.7562) (-259.4177, -103.9169) (-259.2046, -104.0735) (-258.9895, -104.2265) (-258.773, -104.3768) (-258.5553, -104.5251) (-258.3367, -104.6715) (-258.1168, -104.8152) (-257.8944, -104.9538) (-257.6679, -105.0842) (-257.4822, -105.1791) (-257.3398, -105.2438) (-257.2434, -105.2839) (-257.1948, -105.3032) knots -1 -1 -1 -1 -1 -1 -0.98571429 -0.97142857 -0.95714286 -0.94285714 -0.92857143 -0.91428571 -0.9 -0.88571429 -0.87142857 -0.85714286 -0.84285714 -0.82857143 -0.81428571 -0.8 -0.78571429 -0.77142857 -0.75714286 -0.74285714 -0.72857143 -0.71428571 -0.7 -0.68571429 -0.67142857 -0.65714286 -0.64285714 -0.62857143 -0.61428571 -0.6 -0.58571429 -0.57142857 -0.55714286 -0.54285714 -0.52857143 -0.51428571 -0.5 -0.48571429 -0.47142857 -0.45714286 -0.44285714 -0.42857143 -0.41428571 -0.4 -0.38571429 -0.37142857 -0.35714286 -0.34285714 -0.32857143 -0.31428571 -0.3 -0.28571429 -0.27142857 -0.25714286 -0.24285714 -0.22857143 -0.21428571 -0.2 -0.18571429 -0.17142857 -0.15714286 -0.14285714 -0.12857143 -0.11428571 -0.1 -0.08571429 -0.07142857 -0.05714286 -0.04285714 -0.02857143 -0.01428571 0 0 0 0 0 0
  line L7 (-257.1948, -105.3032) -> (-249.6381, -108.3021)
  arc A15 (-248.4946, -110.8399) -> (-249.6381, -108.3021) centre (-250.3759, -110.1611) ccw
  arc A16 (-248.4946, -110.8399) -> (-251.1816, -120.8679) centre (-190.6397, -131.7161) ccw
  arc A17 (-253.4408, -122.494) -> (-251.1816, -120.8679) centre (-253.1502, -120.5152) ccw
  line L8 (-253.4408, -122.494) -> (-261.4845, -121.3128)
  spline S8 degree 5 poles (-261.4845, -121.3128) (-261.5362, -121.3052) (-261.6398, -121.2917) (-261.7955, -121.2765) (-262.0038, -121.2658) (-262.2651, -121.2655) (-262.527, -121.2744) (-262.7893, -121.2889) (-263.0519, -121.3064) (-263.3145, -121.3259) (-263.5772, -121.3478) (-263.8399, -121.3728) (-264.1028, -121.4019) (-264.3657, -121.4356) (-264.6287, -121.474) (-264.8918, -121.5165) (-265.1548, -121.5625) (-265.4178, -121.6115) (-265.6807, -121.6631) (-265.9434, -121.7172) (-266.2061, -121.7739) (-266.4686, -121.8332) (-266.731, -121.8955) (-266.9933, -121.9606) (-267.2554, -122.0285) (-267.5173, -122.0991) (-267.7791, -122.1723) (-268.0406, -122.248) (-268.3019, -122.3259) (-268.563, -122.4063) (-268.8239, -122.4889) (-269.0845, -122.5738) (-269.3448, -122.6611) (-269.6049, -122.7506) (-269.8647, -122.8424) (-270.1243, -122.9365) (-270.3835, -123.0327) (-270.6424, -123.1311) (-270.901, -123.2315) (-271.1593, -123.3341) (-271.4173, -123.4387) (-271.6749, -123.5454) (-271.9321, -123.6541) (-272.1891, -123.7648) (-272.4456, -123.8775) (-272.7018, -123.9922) (-272.9576, -124.1088) (-273.213, -124.2274) (-273.468, -124.3478) (-273.7226, -124.4702) (-273.9768, -124.5944) (-274.2306, -124.7205) (-274.484, -124.8485) (-274.7369, -124.9783) (-274.9894, -125.1099) (-275.2415, -125.2433) (-275.4931, -125.3785) (-275.7442, -125.5154) (-275.9949, -125.6542) (-276.2451, -125.7946) (-276.4949, -125.9368) (-276.7441, -126.0808) (-276.9929, -126.2264) (-277.2412, -126.3738) (-277.489, -126.5228) (-277.7362, -126.6735) (-277.983, -126.8258) (-278.2292, -126.9798) (-278.4749, -127.1355) (-278.7201, -127.2927) (-278.9647, -127.4516) (-279.16, -127.58) (-279.3063, -127.6771) (-279.4036, -127.7421) (-279.4523, -127.7747) knots 0 0 0 0 0 0 0.01428571 0.02857143 0.04285714 0.05714286 0.07142857 0.08571429 0.1 0.11428571 0.12857143 0.14285714 0.15714286 0.17142857 0.18571429 0.2 0.21428571 0.22857143 0.24285714 0.25714286 0.27142857 0.28571429 0.3 0.31428571 0.32857143 0.34285714 0.35714286 0.37142857 0.38571429 0.4 0.41428571 0.42857143 0.44285714 0.45714286 0.47142857 0.48571429 0.5 0.51428571 0.52857143 0.54285714 0.55714286 0.57142857 0.58571429 0.6 0.61428571 0.62857143 0.64285714 0.65714286 0.67142857 0.68571429 0.7 0.71428571 0.72857143 0.74285714 0.75714286 0.77142857 0.78571429 0.8 0.81428571 0.82857143 0.84285714 0.85714286 0.87142857 0.88571429 0.9 0.91428571 0.92857143 0.94285714 0.95714286 0.97142857 0.98571429 1 1 1 1 1 1
  arc A18 (-279.4523, -127.7747) -> (-279.4523, -135.6575) centre (-190.6397, -131.7161) ccw
  spline S9 degree 5 poles (-279.4523, -135.6575) (-279.4036, -135.6901) (-279.3063, -135.7551) (-279.16, -135.8521) (-278.9647, -135.9805) (-278.7201, -136.1394) (-278.4749, -136.2967) (-278.2292, -136.4523) (-277.983, -136.6063) (-277.7362, -136.7587) (-277.489, -136.9094) (-277.2412, -137.0584) (-276.9929, -137.2057) (-276.7441, -137.3514) (-276.4949, -137.4953) (-276.2451, -137.6375) (-275.9949, -137.778) (-275.7442, -137.9167) (-275.4931, -138.0537) (-275.2415, -138.1889) (-274.9894, -138.3223) (-274.7369, -138.4539) (-274.484, -138.5836) (-274.2306, -138.7116) (-273.9768, -138.8377) (-273.7226, -138.9619) (-273.468, -139.0843) (-273.213, -139.2048) (-272.9576, -139.3233) (-272.7018, -139.44) (-272.4456, -139.5546) (-272.1891, -139.6674) (-271.9321, -139.7781) (-271.6749, -139.8868) (-271.4173, -139.9934) (-271.1593, -140.098) (-270.901, -140.2006) (-270.6424, -140.3011) (-270.3835, -140.3994) (-270.1243, -140.4957) (-269.8647, -140.5897) (-269.6049, -140.6815) (-269.3448, -140.7711) (-269.0845, -140.8583) (-268.8239, -140.9433) (-268.563, -141.0259) (-268.3019, -141.1062) (-268.0406, -141.1842) (-267.7791, -141.2598) (-267.5173, -141.333) (-267.2554, -141.4036) (-266.9933, -141.4716) (-266.731, -141.5367) (-266.4686, -141.5989) (-266.2061, -141.6583) (-265.9434, -141.7149) (-265.6807, -141.769) (-265.4178, -141.8206) (-265.1548, -141.8696) (-264.8918, -141.9156) (-264.6287, -141.9581) (-264.3657, -141.9965) (-264.1028, -142.0303) (-263.8399, -142.0594) (-263.5772, -142.0844) (-263.3145, -142.1062) (-263.0519, -142.1258) (-262.7893, -142.1432) (-262.527, -142.1577) (-262.2651, -142.1666) (-262.0038, -142.1663) (-261.7955, -142.1557) (-261.6398, -142.1405) (-261.5362, -142.127) (-261.4845, -142.1194) knots -1 -1 -1 -1 -1 -1 -0.98571429 -0.97142857 -0.95714286 -0.94285714 -0.92857143 -0.91428571 -0.9 -0.88571429 -0.87142857 -0.85714286 -0.84285714 -0.82857143 -0.81428571 -0.8 -0.78571429 -0.77142857 -0.75714286 -0.74285714 -0.72857143 -0.71428571 -0.7 -0.68571429 -0.67142857 -0.65714286 -0.64285714 -0.62857143 -0.61428571 -0.6 -0.58571429 -0.57142857 -0.55714286 -0.54285714 -0.52857143 -0.51428571 -0.5 -0.48571429 -0.47142857 -0.45714286 -0.44285714 -0.42857143 -0.41428571 -0.4 -0.38571429 -0.37142857 -0.35714286 -0.34285714 -0.32857143 -0.31428571 -0.3 -0.28571429 -0.27142857 -0.25714286 -0.24285714 -0.22857143 -0.21428571 -0.2 -0.18571429 -0.17142857 -0.15714286 -0.14285714 -0.12857143 -0.11428571 -0.1 -0.08571429 -0.07142857 -0.05714286 -0.04285714 -0.02857143 -0.01428571 0 0 0 0 0 0
  line L9 (-261.4845, -142.1194) -> (-253.4408, -140.9382)
  arc A19 (-251.1816, -142.5642) -> (-253.4408, -140.9382) centre (-253.1502, -142.9169) ccw
  arc A20 (-251.1816, -142.5642) -> (-248.4946, -152.5923) centre (-190.6397, -131.7161) ccw
  arc A21 (-249.6381, -155.13) -> (-248.4946, -152.5923) centre (-250.3759, -153.2711) ccw
  line L10 (-249.6381, -155.13) -> (-257.1948, -158.129)
  spline S10 degree 5 poles (-257.1948, -158.129) (-257.2434, -158.1482) (-257.3398, -158.1883) (-257.4822, -158.253) (-257.6679, -158.3479) (-257.8944, -158.4783) (-258.1168, -158.617) (-258.3367, -158.7607) (-258.5553, -158.9071) (-258.773, -159.0553) (-258.9895, -159.2056) (-259.2046, -159.3586) (-259.4177, -159.5152) (-259.6285, -159.676) (-259.8371, -159.8407) (-260.0437, -160.009) (-260.2484, -160.1804) (-260.4517, -160.3543) (-260.6536, -160.5304) (-260.8541, -160.7087) (-261.0532, -160.8891) (-261.2509, -161.0717) (-261.447, -161.2568) (-261.6416, -161.4443) (-261.8346, -161.6342) (-262.0262, -161.8264) (-262.2162, -162.0206) (-262.4049, -162.2169) (-262.5922, -162.4151) (-262.7782, -162.6152) (-262.9628, -162.8172) (-263.146, -163.021) (-263.3279, -163.2268) (-263.5083, -163.4344) (-263.6874, -163.6438) (-263.8651, -163.855) (-264.0415, -164.068) (-264.2166, -164.2826) (-264.3903, -164.4989) (-264.5627, -164.7169) (-264.7338, -164.9364) (-264.9036, -165.1576) (-265.072, -165.3804) (-265.2392, -165.6047) (-265.405, -165.8306) (-265.5695, -166.058) (-265.7327, -166.2869) (-265.8946, -166.5173) (-266.0552, -166.7491) (-266.2146, -166.9824) (-266.3726, -167.2171) (-266.5293, -167.4532) (-266.6848, -167.6907) (-266.8389, -167.9296) (-266.9918, -168.1698) (-267.1434, -168.4113) (-267.2937, -168.6542) (-267.4427, -168.8984) (-267.5904, -169.1439) (-267.7369, -169.3907) (-267.8821, -169.6387) (-268.026, -169.888) (-268.1686, -170.1385) (-268.3099, -170.3902) (-268.45, -170.6432) (-268.5888, -170.8973) (-268.7263, -171.1526) (-268.8626, -171.4091) (-268.9975, -171.6668) (-269.1312, -171.9255) (-269.2637, -172.1855) (-269.3686, -172.3943) (-269.4467, -172.5515) (-269.4985, -172.6564) (-269.5244, -172.709) knots 0 0 0 0 0 0 0.01428571 0.02857143 0.04285714 0.05714286 0.07142857 0.08571429 0.1 0.11428571 0.12857143 0.14285714 0.15714286 0.17142857 0.18571429 0.2 0.21428571 0.22857143 0.24285714 0.25714286 0.27142857 0.28571429 0.3 0.31428571 0.32857143 0.34285714 0.35714286 0.37142857 0.38571429 0.4 0.41428571 0.42857143 0.44285714 0.45714286 0.47142857 0.48571429 0.5 0.51428571 0.52857143 0.54285714 0.55714286 0.57142857 0.58571429 0.6 0.61428571 0.62857143 0.64285714 0.65714286 0.67142857 0.68571429 0.7 0.71428571 0.72857143 0.74285714 0.75714286 0.77142857 0.78571429 0.8 0.81428571 0.82857143 0.84285714 0.85714286 0.87142857 0.88571429 0.9 0.91428571 0.92857143 0.94285714 0.95714286 0.97142857 0.98571429 1 1 1 1 1 1
  arc A22 (-269.5244, -172.709) -> (-265.583, -179.5357) centre (-190.6397, -131.7161) ccw
  spline S11 degree 5 poles (-265.583, -179.5357) (-265.5245, -179.5396) (-265.4077, -179.5472) (-265.2325, -179.5581) (-264.9992, -179.5717) (-264.7079, -179.587) (-264.4169, -179.6006) (-264.1263, -179.6125) (-263.8361, -179.6228) (-263.5462, -179.6313) (-263.2567, -179.6382) (-262.9676, -179.6434) (-262.6789, -179.6468) (-262.3907, -179.6486) (-262.1028, -179.6486) (-261.8155, -179.6469) (-261.5285, -179.6434) (-261.2421, -179.6382) (-260.9561, -179.6313) (-260.6706, -179.6225) (-260.3856, -179.6121) (-260.1011, -179.5998) (-259.8172, -179.5857) (-259.5338, -179.5698) (-259.2509, -179.5521) (-258.9687, -179.5326) (-258.687, -179.5113) (-258.4059, -179.4881) (-258.1254, -179.4631) (-257.8456, -179.4362) (-257.5664, -179.4074) (-257.2879, -179.3768) (-257.01, -179.3442) (-256.7329, -179.3097) (-256.4564, -179.2732) (-256.1807, -179.2349) (-255.9058, -179.1945) (-255.6316, -179.1522) (-255.3582, -179.108) (-255.0856, -179.0617) (-254.8138, -179.0134) (-254.5429, -178.963) (-254.2729, -178.9105) (-254.0038, -178.8559) (-253.7356, -178.7991) (-253.4684, -178.7403) (-253.2021, -178.6793) (-252.9368, -178.6161) (-252.6725, -178.5509) (-252.4092, -178.4834) (-252.1471, -178.4136) (-251.8861, -178.3414) (-251.6264, -178.2666) (-251.3681, -178.1893) (-251.111, -178.1095) (-250.8552, -178.0272) (-250.6006, -177.9427) (-250.3472, -177.8559) (-250.0949, -177.7668) (-249.8441, -177.6752) (-249.595, -177.5805) (-249.3481, -177.4822) (-249.1035, -177.3799) (-248.8613, -177.2737) (-248.6213, -177.164) (-248.3828, -177.0516) (-248.1456, -176.9372) (-247.9095, -176.8211) (-247.6751, -176.7024) (-247.4438, -176.5792) (-247.2177, -176.4483) (-247.0427, -176.3349) (-246.9154, -176.2439) (-246.8325, -176.1804) (-246.7915, -176.148) knots -1 -1 -1 -1 -1 -1 -0.98571429 -0.97142857 -0.95714286 -0.94285714 -0.92857143 -0.91428571 -0.9 -0.88571429 -0.87142857 -0.85714286 -0.84285714 -0.82857143 -0.81428571 -0.8 -0.78571429 -0.77142857 -0.75714286 -0.74285714 -0.72857143 -0.71428571 -0.7 -0.68571429 -0.67142857 -0.65714286 -0.64285714 -0.62857143 -0.61428571 -0.6 -0.58571429 -0.57142857 -0.55714286 -0.54285714 -0.52857143 -0.51428571 -0.5 -0.48571429 -0.47142857 -0.45714286 -0.44285714 -0.42857143 -0.41428571 -0.4 -0.38571429 -0.37142857 -0.35714286 -0.34285714 -0.32857143 -0.31428571 -0.3 -0.28571429 -0.27142857 -0.25714286 -0.24285714 -0.22857143 -0.21428571 -0.2 -0.18571429 -0.17142857 -0.15714286 -0.14285714 -0.12857143 -0.11428571 -0.1 -0.08571429 -0.07142857 -0.05714286 -0.04285714 -0.02857143 -0.01428571 0 0 0 0 0 0
  line L11 (-246.7915, -176.148) -> (-240.416, -171.1032)
  arc A23 (-237.6465, -171.3818) -> (-240.416, -171.1032) centre (-239.175, -172.6716) ccw
  arc A24 (-237.6465, -171.3818) -> (-230.3054, -178.7228) centre (-190.6397, -131.7161) ccw
  arc A25 (-230.0268, -181.4924) -> (-230.3054, -178.7228) centre (-231.5952, -180.2513) ccw
  line L12 (-230.0268, -181.4924) -> (-235.0716, -187.8678)
  spline S12 degree 5 poles (-235.0716, -187.8678) (-235.1041, -187.9088) (-235.1675, -187.9918) (-235.2586, -188.119) (-235.3719, -188.2941) (-235.5028, -188.5202) (-235.6261, -188.7515) (-235.7447, -188.9859) (-235.8609, -189.222) (-235.9752, -189.4592) (-236.0876, -189.6976) (-236.1974, -189.9377) (-236.3036, -190.1798) (-236.4058, -190.4244) (-236.5041, -190.6714) (-236.5988, -190.9204) (-236.6905, -191.1713) (-236.7795, -191.4235) (-236.8663, -191.677) (-236.9508, -191.9316) (-237.0331, -192.1874) (-237.113, -192.4444) (-237.1903, -192.7028) (-237.265, -192.9625) (-237.3372, -193.2234) (-237.407, -193.4856) (-237.4745, -193.7488) (-237.5398, -194.0132) (-237.6029, -194.2785) (-237.6639, -194.5447) (-237.7228, -194.812) (-237.7795, -195.0801) (-237.8341, -195.3492) (-237.8866, -195.6192) (-237.937, -195.8901) (-237.9853, -196.1619) (-238.0316, -196.4345) (-238.0759, -196.7079) (-238.1182, -196.9821) (-238.1585, -197.2571) (-238.1969, -197.5328) (-238.2333, -197.8092) (-238.2678, -198.0864) (-238.3004, -198.3642) (-238.3311, -198.6428) (-238.3598, -198.922) (-238.3867, -199.2018) (-238.4118, -199.4823) (-238.4349, -199.7633) (-238.4563, -200.045) (-238.4758, -200.3273) (-238.4935, -200.6101) (-238.5093, -200.8935) (-238.5234, -201.1775) (-238.5357, -201.462) (-238.5462, -201.7469) (-238.5549, -202.0324) (-238.5619, -202.3184) (-238.5671, -202.6049) (-238.5705, -202.8918) (-238.5722, -203.1792) (-238.5722, -203.467) (-238.5705, -203.7553) (-238.567, -204.044) (-238.5619, -204.3331) (-238.555, -204.6226) (-238.5464, -204.9124) (-238.5362, -205.2027) (-238.5242, -205.4933) (-238.5106, -205.7843) (-238.4953, -206.0756) (-238.4818, -206.3089) (-238.4709, -206.484) (-238.4633, -206.6009) (-238.4594, -206.6593) knots 0 0 0 0 0 0 0.01428571 0.02857143 0.04285714 0.05714286 0.07142857 0.08571429 0.1 0.11428571 0.12857143 0.14285714 0.15714286 0.17142857 0.18571429 0.2 0.21428571 0.22857143 0.24285714 0.25714286 0.27142857 0.28571429 0.3 0.31428571 0.32857143 0.34285714 0.35714286 0.37142857 0.38571429 0.4 0.41428571 0.42857143 0.44285714 0.45714286 0.47142857 0.48571429 0.5 0.51428571 0.52857143 0.54285714 0.55714286 0.57142857 0.58571429 0.6 0.61428571 0.62857143 0.64285714 0.65714286 0.67142857 0.68571429 0.7 0.71428571 0.72857143 0.74285714 0.75714286 0.77142857 0.78571429 0.8 0.81428571 0.82857143 0.84285714 0.85714286 0.87142857 0.88571429 0.9 0.91428571 0.92857143 0.94285714 0.95714286 0.97142857 0.98571429 1 1 1 1 1 1
  arc A26 (-238.4594, -206.6593) -> (-231.6326, -210.6007) centre (-190.6397, -131.7161) ccw